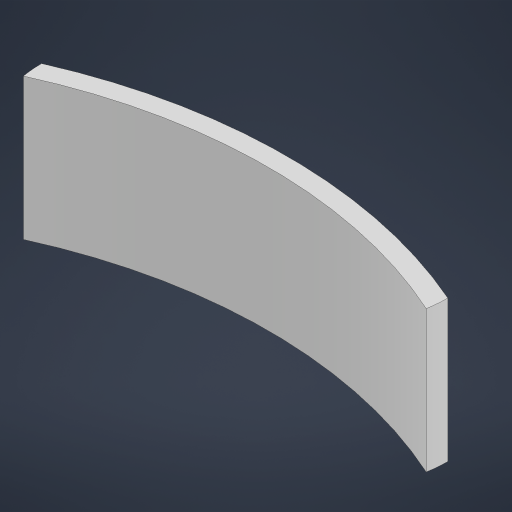
# Autodesk Inventor part: MettalringUnten_v3
Saved by Autodesk Inventor 2023.2 (Build 272271030, 271C)
## iProperties
Created: 2022-10-10
Part Number: MettalringUnten_v3
Material: Generic
Document SubType Name: Modeling
Designer: braun
Density: 1 g/cm^3
Appearance: Default
Author: braun
Autodesk Inventor part; units mm, degrees
ref_plane "YZ Plane" through (0, 0, 0) normal (1, 0, 0) x (0, 1, 0)
ref_plane "XZ Plane" through (0, 0, 0) normal (0, 1, 0) x (-1, 0, 0)
ref_plane "XY Plane" through (0, 0, 0) normal (0, 0, 1) x (1, 0, 0)
sketch "Sketch1" plane through (0, 0, 0) normal (0, 1, 0) x (-1, 0, 0)
  circle A0 centre (0, 0) radius 110 construction
  arc A1 (43.0581, -98.5) -> (-43.0581, -98.5) centre (0, 0) ccw
  line L0 (0, -107.5) -> (0, -98.5) construction
  line L1 (0, -98.5) -> (0, -73.5) construction
  line L2 (0, -98.5) -> (-43.0581, -98.5) construction
  line L3 (0, -98.5) -> (43.0581, -98.5) construction
  line L4 (43.0581, -98.5) -> (-43.0581, -98.5) construction
  line L5 (-18.0581, -73.5) -> (18.0581, -73.5)
  arc A2 (43.0581, -98.5) -> (18.0581, -73.5) centre (18.0581, -98.5) ccw
  arc A3 (-18.0581, -73.5) -> (-43.0581, -98.5) centre (-18.0581, -98.5) ccw
  line L6 (0, 107.5) -> (0, 97.5) construction
  line L7 (0, 97.5) -> (-22.5, 97.5) construction
  line L8 (-22.5, 97.5) -> (-22.5, 82.5) construction
  line L9 (22.5, 82.5) -> (22.5, 97.5) construction
  line L10 (22.5, 90) -> (-22.5, 90) construction
  line L11 (15, 97.5) -> (-15, 97.5)
  line L12 (-15, 82.5) -> (15, 82.5)
  arc A4 (15, 82.5) -> (15, 97.5) centre (15, 90) ccw
  arc A5 (-15, 97.5) -> (-15, 82.5) centre (-15, 90) ccw
  line L13 (22.5, 82.5) -> (17.5, 82.5) construction
  line L14 (17.5, 82.5) -> (17.5, 77.5) construction
  circle A6 centre (17.5, 77.5) radius 1.6
  circle A7 centre (-17.5, 77.5) radius 1.6
  line L15 (-58.3363, 79.5495) -> (-79.5495, 58.3363)
  arc A8 (-47.7297, 68.9429) -> (-58.3363, 79.5495) centre (-53.033, 74.2462) ccw
  arc A9 (-79.5495, 58.3363) -> (-68.9429, 47.7297) centre (-74.2462, 53.033) ccw
  line L16 (-68.9429, 47.7297) -> (-47.7297, 68.9429)
  circle A10 centre (-67.1751, 42.4264) radius 1.6
  circle A11 centre (-42.4264, 67.1751) radius 1.6
  line L17 (-97.5, 15) -> (-97.5, -15)
  arc A12 (-82.5, 15) -> (-97.5, 15) centre (-90, 15) ccw
  arc A13 (-97.5, -15) -> (-82.5, -15) centre (-90, -15) ccw
  line L18 (-82.5, -15) -> (-82.5, 15)
  circle A14 centre (-77.5, -17.5) radius 1.6
  circle A15 centre (-77.5, 17.5) radius 1.6
  line L19 (-79.5495, -58.3363) -> (-58.3363, -79.5495)
  arc A16 (-68.9429, -47.7297) -> (-79.5495, -58.3363) centre (-74.2462, -53.033) ccw
  arc A17 (-58.3363, -79.5495) -> (-47.7297, -68.9429) centre (-53.033, -74.2462) ccw
  line L20 (-47.7297, -68.9429) -> (-68.9429, -47.7297)
  circle A18 centre (-42.4264, -67.1751) radius 1.6
  circle A19 centre (-67.1751, -42.4264) radius 1.6
  line L21 (-15, -97.5) -> (15, -97.5)
  arc A20 (-15, -82.5) -> (-15, -97.5) centre (-15, -90) ccw
  arc A21 (15, -97.5) -> (15, -82.5) centre (15, -90) ccw
  line L22 (15, -82.5) -> (-15, -82.5)
  circle A22 centre (17.5, -77.5) radius 1.6
  circle A23 centre (-17.5, -77.5) radius 1.6
  line L23 (58.3363, -79.5495) -> (79.5495, -58.3363)
  arc A24 (47.7297, -68.9429) -> (58.3363, -79.5495) centre (53.033, -74.2462) ccw
  arc A25 (79.5495, -58.3363) -> (68.9429, -47.7297) centre (74.2462, -53.033) ccw
  line L24 (68.9429, -47.7297) -> (47.7297, -68.9429)
  circle A26 centre (67.1751, -42.4264) radius 1.6
  circle A27 centre (42.4264, -67.1751) radius 1.6
  line L25 (97.5, -15) -> (97.5, 15)
  arc A28 (82.5, -15) -> (97.5, -15) centre (90, -15) ccw
  arc A29 (97.5, 15) -> (82.5, 15) centre (90, 15) ccw
  line L26 (82.5, 15) -> (82.5, -15)
  circle A30 centre (77.5, 17.5) radius 1.6
  circle A31 centre (77.5, -17.5) radius 1.6
  line L27 (79.5495, 58.3363) -> (58.3363, 79.5495)
  arc A32 (68.9429, 47.7297) -> (79.5495, 58.3363) centre (74.2462, 53.033) ccw
  arc A33 (58.3363, 79.5495) -> (47.7297, 68.9429) centre (53.033, 74.2462) ccw
  line L28 (47.7297, 68.9429) -> (68.9429, 47.7297)
  circle A34 centre (42.4264, 67.1751) radius 1.6
  circle A35 centre (67.1751, 42.4264) radius 1.6
  line L29 (58.3363, -58.3363) -> (51.2652, -51.2652) construction
  line L30 (40.6586, -61.8718) -> (61.8718, -40.6586)
  arc A36 (40.6586, -61.8718) -> (44.5267, -89.5398) centre (53.033, -74.2462) ccw
  arc A37 (89.5398, -44.5267) -> (61.8718, -40.6586) centre (74.2462, -53.033) ccw
  line L31 (0, -73.5) -> (0, -66.5) construction
  arc A38 (44.5267, 89.5398) -> (40.6586, 61.8718) centre (53.033, 74.2462) ccw
  line L32 (61.8718, 40.6586) -> (40.6586, 61.8718)
  arc A39 (61.8718, 40.6586) -> (89.5398, 44.5267) centre (74.2462, 53.033) ccw
  arc A40 (-89.5398, 44.5267) -> (-61.8718, 40.6586) centre (-74.2462, 53.033) ccw
  line L33 (-40.6586, 61.8718) -> (-61.8718, 40.6586)
  arc A41 (-40.6586, 61.8718) -> (-44.5267, 89.5398) centre (-53.033, 74.2462) ccw
  arc A42 (-44.5267, -89.5398) -> (-40.6586, -61.8718) centre (-53.033, -74.2462) ccw
  line L34 (-61.8718, -40.6586) -> (-40.6586, -61.8718)
  arc A43 (-61.8718, -40.6586) -> (-89.5398, -44.5267) centre (-74.2462, -53.033) ccw
  arc A44 (89.5398, -44.5267) -> (89.5398, 44.5267) centre (0, 0) ccw
  arc A45 (44.5267, 89.5398) -> (-44.5267, 89.5398) centre (0, 0) ccw
  arc A46 (-89.5398, 44.5267) -> (-89.5398, -44.5267) centre (0, 0) ccw
  line L35 (43.0581, -98.5) -> (48.0581, -98.5) construction
  line L36 (48.0581, -98.5) -> (48.0581, -88.5) construction
  circle A47 centre (48.0581, -88.5) radius 1.6
  circle A48 centre (-48.0581, -88.5) radius 1.6
  line L37 (18.0581, -66.5) -> (-18.0581, -66.5)
  arc A49 (17.5, -66.5) -> (43.0581, -59.4724) centre (19.5145, -23.8377) ccw
  arc A50 (-44.5267, -58.0038) -> (-18.0581, -66.5) centre (-19.5089, -25.5422) ccw
  arc A51 (-48.0581, -88.5) -> (-42.4264, -67.1751) centre (-60.4397, -73.8241) ccw construction
  arc A52 (-48.0581, -88.5) -> (-42.4264, -67.1751) centre (-60.4397, -73.8241) ccw construction
  arc A53 (-44.9367, -92.1998) -> (-37.8853, -65.499) centre (-60.4397, -73.8241) ccw
  arc A54 (-51.1795, -84.8002) -> (-46.9675, -68.8513) centre (-60.4397, -73.8241) ccw
  arc A55 (-51.1795, -84.8002) -> (-44.9367, -92.1998) centre (-48.0581, -88.5) ccw
  arc A56 (-37.8853, -65.499) -> (-46.9675, -68.8513) centre (-42.4264, -67.1751) ccw
  line L38 (42.4264, 67.1751) -> (67.1751, 42.4264) construction
  line L39 (45.9619, 70.7107) -> (70.7107, 45.9619)
  line L40 (63.6396, 38.8909) -> (38.8909, 63.6396)
  arc A57 (45.9619, 70.7107) -> (38.8909, 63.6396) centre (42.4264, 67.1751) ccw
  arc A58 (63.6396, 38.8909) -> (70.7107, 45.9619) centre (67.1751, 42.4264) ccw
  line L41 (-42.4264, 67.1751) -> (-67.1751, 42.4264) construction
  line L42 (-45.9619, 70.7107) -> (-70.7107, 45.9619)
  line L43 (-63.6396, 38.8909) -> (-38.8909, 63.6396)
  arc A59 (-38.8909, 63.6396) -> (-45.9619, 70.7107) centre (-42.4264, 67.1751) ccw
  arc A60 (-70.7107, 45.9619) -> (-63.6396, 38.8909) centre (-67.1751, 42.4264) ccw
  line L44 (-42.4264, 67.1751) -> (42.4264, 67.1751) construction
  line L45 (-42.4264, 62.1751) -> (42.4264, 62.1751)
  line L46 (42.4264, 72.1751) -> (-42.4264, 72.1751)
  arc A61 (-42.4264, 72.1751) -> (-42.4264, 62.1751) centre (-42.4264, 67.1751) ccw
  arc A62 (42.4264, 62.1751) -> (42.4264, 72.1751) centre (42.4264, 67.1751) ccw
  line L47 (37.0252, 67.1751) -> (33.0252, 67.1751) construction
  line L48 (33.0252, 67.1751) -> (32.0252, 67.1751) construction
  line L49 (31.0252, 70.4251) -> (31.0252, 63.9251)
  line L50 (31.0252, 63.9251) -> (33.0252, 63.9251)
  line L51 (33.0252, 63.9251) -> (33.0252, 70.4251)
  line L52 (33.0252, 70.4251) -> (31.0252, 70.4251)
  line L53 (31.0252, 70.4251) -> (33.0252, 63.9251) construction
  line L54 (31.0252, 63.9251) -> (33.0252, 70.4251) construction
  line L55 (0, 67.1751) -> (0, 56.5088) construction
  line L56 (-31.0252, 70.4251) -> (-31.0252, 63.9251)
  line L57 (-31.0252, 63.9251) -> (-33.0252, 63.9251)
  line L58 (-33.0252, 63.9251) -> (-33.0252, 70.4251)
  line L59 (-33.0252, 70.4251) -> (-31.0252, 70.4251)
  arc A63 (-43.0581, -98.5) -> (43.0581, -98.5) centre (0, 0) ccw
  line L60 (0, -107.5) -> (0, -103.5)
  arc A64 (-41.4559, -94.8349) -> (41.4559, -94.8349) centre (0, 0) ccw
  arc A65 (41.4559, -94.8349) -> (42.6996, -94.2815) centre (0, 0) ccw
  arc A66 (-42.6996, -94.2815) -> (-41.4559, -94.8349) centre (0, 0) ccw
  point P0 (0, 90)
  point P1 (-45.9619, 70.7107)
  point P2 (-82.5, 17.5)
  point P3 (-70.7107, -45.9619)
  point P4 (-17.5, -82.5)
  point P5 (45.9619, -70.7107)
  point P6 (82.5, -17.5)
  point P7 (70.7107, 45.9619)
  point P8 (35.7159, -76.7698)
  point P9 (-37.9023, -65.4535)
  point P10 (-39.0971, -63.6613)
  point P11 (-46.4221, -70.7043)
  point P12 (-46.8673, -78.5164)
  point P13 (0, -44.5267)
  point P14 (0, 35.7016)
  point P15 (54.8008, 54.8008)
  point P16 (-54.8008, 54.8008)
  point P17 (40.3553, 62.1751)
  point P18 (40.6586, 61.8718)
  point P19 (-47.7297, 68.9429)
  point P20 (-68.9429, 47.7297)
  point P21 (-61.8718, 40.6586)
  point P22 (-40.3553, 62.1751)
  dimension "d0" = 220
  dimension "d1" = 215
  dimension "d2" = 9
  dimension "d3" = 25
  dimension "d4" = 10
  dimension "d5" = 22.5
  dimension "d6" = 15
  dimension "d7" = 45
  dimension "d8" = 5
  dimension "d9" = 5
  dimension "d10" = 3.2
  dimension "d15" = 86.1162
  dimension "d16" = 45
  dimension "d19" = 360
  dimension "d22" = 10
  dimension "d23" = 7
  dimension "d26" = 360
  dimension "d33" = 5
  dimension "d34" = 10
  dimension "d35" = 3.2
  dimension "d68" = 4
  dimension "d69" = 1
  dimension "d70" = 6.5
  dimension "d71" = 2
  dimension "d123" = 4
  constraints: 132 end point, 107 point on circle, 67 centre point, 24 tangent, 23 point on line, 10 midpoint, 6 parallel, 6 symmetric about line, 5 coincident, 5 vertical, 4 perpendicular, 3 horizontal, 2 concentric, 1 collinear, 160 other
  measures "d0" diameter of A0
  measures "d1" diameter of A1
  measures "d2" distance of L0.start L0.end
  measures "d3" distance of L0.end L1.end
  measures "d4" distance of L6.start L6.end
  measures "d5" distance of L6.end L7.end
  measures "d6" distance of L7.end L8.end
  measures "d7" distance of L8.end L9.start
  measures "d8" distance of L9.start L13.end
  measures "d9" distance of L13.end L14.end
  measures "d10" diameter of A6
  measures "d15" distance of L3.end L2.end
  measures "d16" distance of L10.start L10.end
  measures "d22" distance of L29.start L29.end
  measures "d23" distance of L1.end L31.end
  measures "d33" distance of L3.end L35.end
  measures "d34" distance of L35.end L36.end
  measures "d35" diameter of A47
  measures "d68" distance of L47.start L47.end
  measures "d69" distance of L47.end L48.end
  measures "d70" distance of L49.start L49.end
  measures "d71" distance of L50.end L49.end
  measures "d123" distance of L0.start L60.end
ref_plane "Work Plane4" through (0, 0, -44.5267) normal (1, 0, 0) x (0, 0.9903099, -0.1388753)
extrude "Extrusion13" add sketch "Sketch1" against normal blind 30 contours A63 L60 A64 A65 A2 | A3 A66 A64 L60 A63
body "Solid4"
